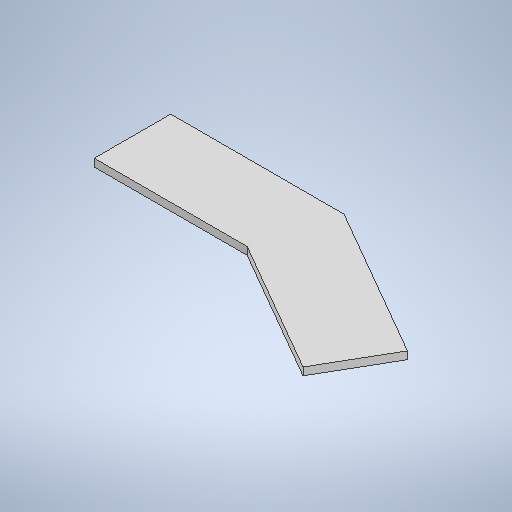
# Autodesk Inventor part: 150degreesidebracker
Saved by Autodesk Inventor 2025.2 (Build 292293000, 293)
## iProperties
Created: 2026-03-25
Part Number: 150degreesidebracker
Material: Generic
Document SubType Name: Modeling
Designer: hp
Density: 1 g/cm^3
Appearance: Default
Author: hp
Autodesk Inventor part; units mm, degrees
ref_plane "YZ Plane" through (0, 0, 0) normal (1, 0, 0) x (0, 1, 0)
ref_plane "XZ Plane" through (0, 0, 0) normal (0, 1, 0) x (-1, 0, 0)
ref_plane "XY Plane" through (0, 0, 0) normal (0, 0, 1) x (1, 0, 0)
sketch "Sketch1" plane through (0, 0, 0) normal (0, 1, 0) x (-1, 0, 0)
  line L0 (0, 0) -> (-34.641, 20)
  line L1 (0, 0) -> (40, 0) construction
  line L2 (-34.641, 20) -> (-44.641, 2.6795)
  line L3 (-44.641, 2.6795) -> (-10, -17.3205)
  line L4 (0, 0) -> (40, 0)
  line L5 (40, 0) -> (40, -20)
  line L6 (40, -20) -> (-5.359, -20)
  line L7 (-5.359, -20) -> (-10, -17.3205)
  dimension "d0" = 40
  dimension "d1" = 150
  dimension "d2" = 20
  dimension "d3" = 40
  dimension "d4" = 20
  constraints: 16 end point, 4 perpendicular, 1 collinear, 1 equal length, 1 horizontal
  measures "d0" distance of L0.start L0.end
  measures "d1" angle of L1 L0
  measures "d2" distance of L0.end L2.end
  measures "d3" distance of L0.start L1.end
  measures "d4" distance of L1.end L5.end
extrude "Extrusion1" add sketch "Sketch1" along normal blind 2
body "Solid1"
